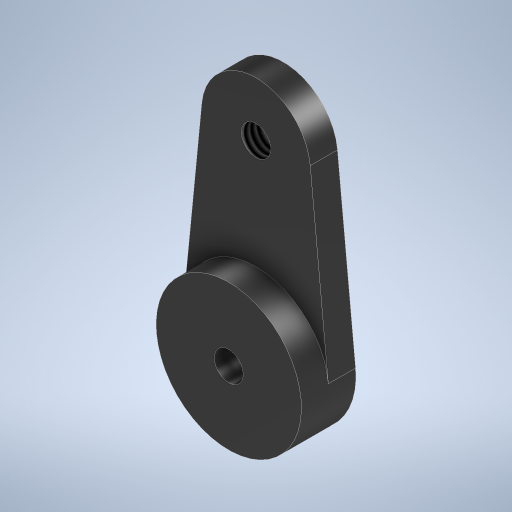
# Autodesk Inventor part: LongCrankFrameBasis
Saved by Autodesk Inventor 2024.2 (Build 282272000, 272)
## iProperties
Created: 2024-01-04
Part Number: LongCrankFrameBasis
Material: Aluminum 7075
Document SubType Name: Modeling
Designer: Masato Kubotera
Density: 2.81 g/cm^3
Appearance: Glossy - Black
Vendor: meviy
Mass: 4.45971 g
Surface Area: 13.3762 cm^2
Volume: 1.58709 cm^3
Author: Masato Kubotera
Autodesk Inventor part; units mm, degrees
ref_plane "YZ Plane" through (0, 0, 0) normal (1, 0, 0) x (0, 1, 0)
ref_plane "XZ Plane" through (0, 0, 0) normal (0, 1, 0) x (-1, 0, 0)
ref_plane "XY Plane" through (0, 0, 0) normal (0, 0, 1) x (1, 0, 0)
sketch "Sketch1" plane through (0, 0, 0) normal (1, 0, 0) x (0, 1, 0)
  circle A0 centre (0, 0) radius 8
  line L0 (0, 20) -> (0, 0) construction
  arc A1 (5.9699, 20.6) -> (-5.9699, 20.6) centre (0, 20) ccw
  line L1 (-7.9599, 0.8) -> (-5.9699, 20.6)
  line L2 (7.9599, 0.8) -> (5.9699, 20.6)
  line L3 (-5.3312, 5.9647) -> (7.8312, -1.6346) construction
  line L4 (5.3312, -5.9647) -> (-7.8312, 1.6346) construction
  line L5 (-6.9282, 4) -> (6.9282, -4) construction
  line L6 (-5.3116, 5.9823) -> (7.8366, -1.6088)
  line L7 (-7.8366, 1.6088) -> (5.3116, -5.9823)
  line L8 (5.3312, 5.9647) -> (-7.8312, -1.6346) construction
  line L9 (-5.3312, -5.9647) -> (7.8312, 1.6346) construction
  line L10 (6.9282, 4) -> (-6.9282, -4) construction
  line L11 (5.3116, 5.9823) -> (-7.8366, -1.6088)
  line L12 (7.8366, 1.6088) -> (-5.3116, -5.9823)
  line L13 (-7.5911, 2.525) -> (7.5911, 2.525)
  line L14 (-7.5993, 2.5) -> (7.5993, 2.5) construction
  line L15 (-8, 0) -> (8, 0) construction
  line L16 (-7.5911, -2.525) -> (7.5911, -2.525)
  line L17 (-7.5993, -2.5) -> (7.5993, -2.5) construction
  point P0 (7.9599, 0.8)
  point P1 (-5.3116, -5.9823)
  point P2 (0, -2.9156)
  point P3 (5.3116, -5.9823)
  point P4 (5.05, 0)
  point P5 (7.8366, 1.6088)
  point P6 (5.3116, 5.9823)
  point P7 (0, 2.9156)
  point P8 (-7.8366, 1.6088)
  point P9 (-5.05, 0)
  point P10 (-7.8366, -1.6088)
  dimension "d0" = 16
  dimension "d1" = 20
  dimension "d2" = 12
  dimension "d28" = 60
  dimension "d29" = 5
  dimension "d30" = 0.025
  dimension "d31" = 5
  dimension "d32" = 0.025
  constraints: 36 end point, 18 symmetric about line, 3 coincident, 3 horizontal, 2 midpoint, 2 parallel, 2 point on circle, 1 centre point, 1 tangent, 1 vertical, 19 other
  measures "d1" distance of L0.start L0.end
  measures "d2" diameter of A1
  measures "d28" angle of L5 L0
  measures "d29" distance between parallel lines of L4 L3
  measures "d30" distance between parallel lines of L3 L6
  measures "d31" distance between parallel lines of L17 L14
  measures "d32" distance between parallel lines of L14 L13
extrude "Extrusion1" add sketch "Sketch1" against normal blind 6
extrude "Extrusion2" cut sketch "Sketch1" against normal blind 3 contours A0 L1 A1 L2
hole "M4" at (0, 0, 20) direction (-1, 0, 0) diameter 3.242 end through all thread size "M4x0.7" class "6H" standard "ANSI Metric M Profile"
hole "Phi3.2" at (0, 0, 0) direction (-1, 0, 0) diameter 3.2 end through all
equation "\"d31\" = d29"
equation "\"d32\" = d30"
body "Solid1"
